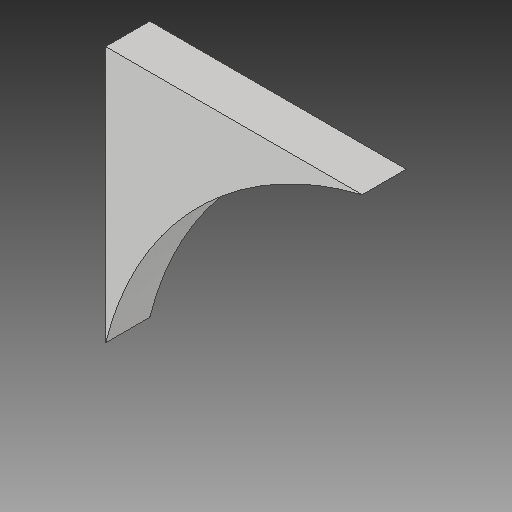
# Autodesk Inventor part: Corner
Saved by Autodesk Inventor 2019.3 (Build 233278000, 278)
## iProperties
Created: 2020-08-27
Part Number: Corner
Material: Generisch
Document SubType Name: Modeling
Designer: Nicolas Frick
Density: 1 g/cm^3
Appearance: Vorgabe
Author: Nicolas Frick
Autodesk Inventor part; units mm, degrees
ref_plane "YZ Plane" through (0, 0, 0) normal (1, 0, 0) x (0, 1, 0)
ref_plane "XZ Plane" through (0, 0, 0) normal (0, 1, 0) x (-1, 0, 0)
ref_plane "XY Plane" through (0, 0, 0) normal (0, 0, 1) x (1, 0, 0)
sketch "Skizze1" plane through (0, 0, 0) normal (0, 0, 1) x (1, 0, 0)
  line L0 (-901.5, -442.5) -> (-901.5, 442.5) construction
  line L1 (-901.5, 442.5) -> (901.5, 442.5) construction
  line L2 (901.5, 442.5) -> (901.5, -442.5) construction
  line L3 (901.5, -442.5) -> (-901.5, -442.5) construction
  line L4 (914, 455) -> (-914, 455) construction
  line L5 (-914, 455) -> (-914, -455) construction
  line L6 (-914, -455) -> (914, -455) construction
  line L7 (914, -455) -> (914, 455) construction
  line L8 (-901.5, 442.5) -> (-808.5, 442.5)
  line L9 (-901.5, 442.5) -> (-901.5, 349.5)
  arc A0 (-808.5, 442.5) -> (-901.5, 349.5) centre (-777.5545, 318.5545) ccw
  point P0 (0, 0)
  dimension "d0" = 93
  dimension "d1" = 93
  constraints: 4 end point, 2 point on circle, 2 point on line, 1 centre point
  measures "d0" distance of L0.end L8.end
  measures "d1" distance of L0.end L9.end
ref_plane "Arbeitsebene1" through (-914, -455, 16) normal (0, 0, 1) x (1, 0, 0)
extrude "Extrusion1" add sketch "Skizze1" along normal up to surface (16 mm away)
